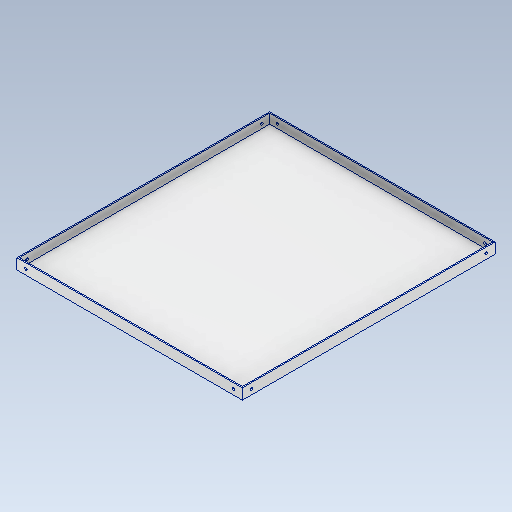
# Autodesk Inventor part: Bandeja
Saved by Autodesk Inventor 2020 (Build 240168000, 168)
## iProperties
Created: 2020-05-08
Part Number: Bandeja
Material: Aluminum 6061
Document SubType Name: Modeling
Designer: Pipi
Density: 2.7 g/cm^3
Appearance: Aluminum - Flat
Author: Pipi
Autodesk Inventor part; units mm, degrees
ref_plane "YZ Plane" through (0, 0, 0) normal (1, 0, 0) x (0, 1, 0)
ref_plane "XZ Plane" through (0, 0, 0) normal (0, 1, 0) x (-1, 0, 0)
ref_plane "XY Plane" through (0, 0, 0) normal (0, 0, 1) x (1, 0, 0)
sketch "Boceto1" plane through (0, 0, 0) normal (0, 1, 0) x (-1, 0, 0)
  line L0 (9.2464, 12.6324) -> (9.2464, -413.3676)
  line L1 (9.2464, -413.3676) -> (-370.7536, -413.3676)
  line L2 (-370.7536, -413.3676) -> (-370.7536, 12.6324)
  line L3 (-370.7536, 12.6324) -> (9.2464, 12.6324)
  line L4 (9.2464, 12.6324) -> (9.2464, 10.6324)
  line L5 (9.2464, 10.6324) -> (-370.7536, 10.6324)
  line L6 (-370.7536, 10.6324) -> (-368.7536, 10.6324)
  line L7 (-368.7536, 10.6324) -> (-368.7536, -413.3676)
  line L8 (-368.7536, -413.3676) -> (-368.7536, -411.3676)
  line L9 (-368.7536, -411.3676) -> (9.2464, -411.3676)
  line L10 (9.2464, -411.3676) -> (7.2464, -411.3676)
  line L11 (9.2464, 10.6324) -> (7.2464, 10.6324)
  line L12 (7.2464, 10.6324) -> (7.2464, -411.3676)
  point P0 (0, 0)
  dimension "d0" = 426
  dimension "d1" = 380
  dimension "d2" = 2
  dimension "d3" = 2
  dimension "d4" = 2
  dimension "d5" = 2
  dimension "d6" = 2
  constraints: 26 end point, 8 point on line, 5 perpendicular, 1 parallel, 1 vertical
  measures "d0" distance of L0.start L0.end
  measures "d1" distance of L0.end L1.end
  measures "d2" distance of L0.start L4.end
  measures "d3" distance of L5.end L6.end
  measures "d4" distance of L7.end L8.end
  measures "d5" distance of L9.end L10.end
  measures "d6" distance of L4.end L11.end
extrude "Extrusión1" add sketch "Boceto1" along normal blind 2 contours L12 L9 L7 L5
extrude "Extrusión2" add sketch "Boceto1" along normal blind 18 contours L0 L5 L2 L3 | L0 L9 L12 L5 | L0 L1 L7 L9 | L5 L7 L1 L2
sketch "Boceto2" plane through (-9.2464, 0, 12.6324) normal (0, 0, 1) x (1, 0, 0)
  point P0 (9.2464, 0)
sketch "Boceto3" plane through (-9.2464, 0, 12.6324) normal (0, 0, 1) x (1, 0, 0)
  point P0 (9.2464, 0)
sketch "Boceto7" plane through (370.7536, 0, 12.6324) normal (1, 0, 0) x (0, 0, -1)
  line L0 (0, 0) -> (0, 18) projected
  line L1 (0, 9) -> (425.996, 9)
  line L2 (2, 2) -> (424, 2) projected
  circle A0 centre (15, 9) radius 2.125
  circle A1 centre (411, 9) radius 2.125
  line L3 (426, 0) -> (426, 18) projected
  point P0 (12.6324, 0)
  dimension "d29" = 4.25
  dimension "d30" = 4.25
  dimension "d31" = 15
  dimension "d32" = 15
  constraints: 2 centre point, 2 end point, 2 point on line, 1 midpoint, 1 parallel
  measures "d29" diameter of A0
  measures "d30" diameter of A1
  measures "d31" distance of A0.centre L1.start
  measures "d32" distance from line of L3 A1.centre
sketch "Boceto8" plane through (-9.2464, 0, 12.6324) normal (0, 0, 1) x (1, 0, 0)
  line L0 (0, 0) -> (0, 18) projected
  line L1 (0, 9) -> (380, 9.366)
  line L2 (380, 0) -> (380, 18) projected
  circle A0 centre (365, 9.3516) radius 2.125
  circle A1 centre (15, 9.0201) radius 2.125
  point P0 (9.2464, 0)
  dimension "d33" = 4.25
  dimension "d34" = 4.25
  dimension "d35" = 15
  dimension "d36" = 15
  constraints: 2 centre point, 2 end point, 2 point on line, 1 midpoint
  measures "d33" diameter of A0
  measures "d34" diameter of A1
  measures "d35" distance from line of L0 A1.centre
  measures "d36" distance from line of L2 A0.centre
extrude "Extrusión6" cut sketch "Boceto8" against normal blind 1000
extrude "Extrusión7" cut sketch "Boceto7" against normal blind 1000
